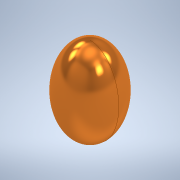
# Autodesk Inventor part: Ei
Saved by Autodesk Inventor 2020 (Build 240168000, 168)
## iProperties
Created: 2021-05-05
Part Number: Ei
Material: Gold
Document SubType Name: Modeling
Designer: Julian Uhl
Density: 19.3 g/cm^3
Appearance: Metall - 1600F (heiß)
Author: Julian Uhl
Autodesk Inventor part; units mm, degrees
ref_plane "YZ Plane" through (0, 0, 0) normal (1, 0, 0) x (0, 1, 0)
ref_plane "XZ Plane" through (0, 0, 0) normal (0, 1, 0) x (-1, 0, 0)
ref_plane "XY Plane" through (0, 0, 0) normal (0, 0, 1) x (1, 0, 0)
sketch "Skizze2" plane through (0, 0, 0) normal (0, 0, 1) x (1, 0, 0)
  line L0 (0, 42) -> (0, -42) projected
  line L1 (-28, 0) -> (28, 0) projected
  line L2 (-28, 0) -> (28, 0) projected
  line L3 (0, -42) -> (0, 42) projected
  ellipse E0 centre (0, 0) end of major axis (-20, 0) minor radius 30
  point P0 (0, 30)
  point P1 (0, -30)
  dimension "d0" = 20
  dimension "d1" = 30
  constraints: 1 coincident, 2 other
revolve "Umdrehung1" add sketch "Skizze2" angle 360 about axis through (0, 0, 0) along (0, -1, 0) picked at (2.0342, 19.5231) picked at (2.5179, -19.2593) contours E0 L1 L0 | L1 E0 L0
